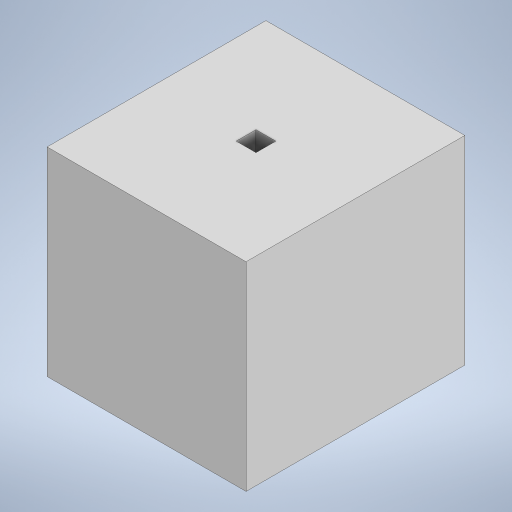
# Autodesk Inventor part: four-blocks
Saved by Autodesk Inventor 2023 (Build 270158000, 158)
## iProperties
Created: 2023-05-03
Part Number: four-blocks
Material: Generic
Document SubType Name: Modeling
Designer: Anya
Density: 1 g/cm^3
Appearance: Default
Author: Anya
Autodesk Inventor part; units mm, degrees
ref_plane "YZ Plane" through (0, 0, 0) normal (1, 0, 0) x (0, 1, 0)
ref_plane "XZ Plane" through (0, 0, 0) normal (0, 1, 0) x (-1, 0, 0)
ref_plane "XY Plane" through (0, 0, 0) normal (0, 0, 1) x (1, 0, 0)
sketch "Sketch4" plane through (0, 0, 0) normal (0, 1, 0) x (-1, 0, 0)
  line L0 (100, 110) -> (-100, 110)
  line L1 (-100, 110) -> (-100, 10)
  line L2 (-100, 10) -> (100, 10)
  line L3 (100, 10) -> (100, 110)
  line L4 (100, 110) -> (-100, 10) construction
  line L5 (-100, 110) -> (100, 10) construction
  line L6 (100, 110) -> (-100, 110)
  line L7 (-100, 110) -> (-100, 10)
  line L8 (-100, 10) -> (100, 10)
  line L9 (100, 10) -> (100, 110)
  line L10 (100, 110) -> (-100, 10) construction
  line L11 (-100, 110) -> (100, 10) construction
  line L12 (100, -10) -> (-100, -10)
  line L13 (-100, -10) -> (-100, -110)
  line L14 (-100, -110) -> (100, -110)
  line L15 (100, -110) -> (100, -10)
  line L16 (100, -10) -> (-100, -110) construction
  line L17 (-100, -10) -> (100, -110) construction
  point P0 (0, 0)
  point P1 (0, 60)
  point P2 (0, 60)
  point P3 (0, -60)
  dimension "d8" = 200
  dimension "d9" = 100
  dimension "d12" = 200
  dimension "d13" = 100
  dimension "d14" = 200
  dimension "d15" = 100
  constraints: 36 end point, 6 midpoint, 6 parallel, 3 horizontal, 3 perpendicular
  measures "d8" distance of L0.start L0.end
  measures "d9" distance of L2.end L0.start
  measures "d12" distance of L10.start L7.start
  measures "d13" distance of L9.start L10.start
  measures "d14" distance of L16.start L13.start
  measures "d15" distance of L15.start L16.start
sketch "Sketch5" plane through (0, 0, 0) normal (0, 1, 0) x (-1, 0, 0)
  line L0 (100, 10) -> (10, 10)
  line L1 (10, 10) -> (10, -10)
  line L2 (10, -10) -> (100, -10)
  line L3 (100, -10) -> (100, 10)
  line L4 (100, 10) -> (10, -10) construction
  line L5 (10, 10) -> (100, -10) construction
  line L6 (100, 10) -> (10, 10)
  line L7 (10, 10) -> (10, -10)
  line L8 (10, -10) -> (100, -10)
  line L9 (100, -10) -> (100, 10)
  line L10 (100, 10) -> (10, -10) construction
  line L11 (10, 10) -> (100, -10) construction
  line L12 (-10, 10) -> (-100, 10)
  line L13 (-100, 10) -> (-100, -10)
  line L14 (-100, -10) -> (-10, -10)
  line L15 (-10, -10) -> (-10, 10)
  line L16 (-10, 10) -> (-100, -10) construction
  line L17 (-100, 10) -> (-10, -10) construction
  point P0 (0, 0)
  point P1 (55, 0)
  point P2 (55, 0)
  point P3 (-55, 0)
  dimension "d10" = 90
  dimension "d11" = 20
  dimension "d16" = 90
  dimension "d17" = 20
  dimension "d18" = 90
  dimension "d19" = 20
  constraints: 36 end point, 6 midpoint, 6 parallel, 3 horizontal, 3 perpendicular
  measures "d10" distance of L0.start L0.end
  measures "d11" distance of L2.end L0.start
  measures "d16" distance of L6.start L6.end
  measures "d17" distance of L8.end L6.start
  measures "d18" distance of L12.start L12.end
  measures "d19" distance of L14.end L12.start
extrude "Extrusion1" add sketch "Sketch4" along normal mid plane 200
extrude "Extrusion2" add sketch "Sketch5" along normal mid plane 200
body "Solid1"
